Autodesk Inventor part; units mm, degrees
(part 4 of 4)
  arc A540 (15.9898, 14.9832) -> (15.5153, 14.8775) centre (17.401, 7.5282) ccw projected
  arc A541 (15.5153, 14.8775) -> (15.1369, 14.7679) centre (17.1075, 8.6707) ccw projected
  arc A542 (15.1369, 14.7679) -> (14.8419, 14.6628) centre (16.7577, 9.7513) ccw projected
  arc A543 (14.8419, 14.6628) -> (14.619, 14.9696) centre (-0.9435, 3.4284) ccw projected
  arc A544 (14.619, 14.9696) -> (14.8101, 15.2177) centre (10.5399, 18.3094) ccw projected
  arc A545 (14.8101, 15.2177) -> (15.0312, 15.5438) centre (9.6202, 18.976) ccw projected
  arc A546 (15.0312, 15.5438) -> (15.2784, 15.9624) centre (8.6244, 19.6082) ccw projected
  arc A547 (15.2784, 15.9624) -> (15.0311, 16.2761) centre (-0.9435, 3.4284) ccw projected
  arc A548 (15.0311, 16.2761) -> (14.5663, 16.1335) centre (17.0228, 8.9549) ccw projected
  arc A549 (14.5663, 16.1335) -> (14.1976, 15.9946) centre (16.6405, 10.0708) ccw projected
  arc A550 (14.1976, 15.9946) -> (13.9118, 15.8667) centre (16.2071, 11.1207) ccw projected
  arc A551 (13.9118, 15.8667) -> (13.6655, 16.1551) centre (-0.9435, 3.4284) ccw projected
  arc A552 (13.6655, 16.1551) -> (13.8365, 16.4174) centre (9.3369, 19.1645) ccw projected
  arc A553 (13.8365, 16.4174) -> (14.0314, 16.7598) centre (8.3678, 19.7569) ccw projected
  arc A554 (14.0314, 16.7598) -> (14.2449, 17.1965) centre (7.3254, 20.309) ccw projected
  arc A555 (14.2449, 17.1965) -> (13.9738, 17.4899) centre (-0.9435, 3.4284) ccw projected
  arc A556 (13.9738, 17.4899) -> (13.5217, 17.3113) centre (16.5338, 10.3475) ccw projected
  arc A557 (13.5217, 17.3113) -> (13.165, 17.1438) centre (16.0652, 11.43) ccw projected
  arc A558 (13.165, 17.1438) -> (12.8901, 16.9939) centre (15.5507, 12.4426) ccw projected
  arc A559 (12.8901, 16.9939) -> (12.6219, 17.2621) centre (-0.9435, 3.4284) ccw projected
  arc A560 (12.6219, 17.2621) -> (12.7719, 17.537) centre (8.0706, 19.9226) ccw projected
  arc A561 (12.7719, 17.537) -> (12.9393, 17.8936) centre (7.058, 20.4371) ccw projected
  arc A562 (12.9393, 17.8936) -> (13.1179, 18.3458) centre (5.9755, 20.9058) ccw projected
  arc A563 (13.1179, 18.3458) -> (12.8246, 18.6169) centre (-0.9435, 3.4284) ccw projected
  arc A564 (12.8246, 18.6169) -> (12.3878, 18.4034) centre (15.9371, 11.6974) ccw projected
  arc A565 (12.3878, 18.4034) -> (12.0454, 18.2085) centre (15.3849, 12.7398) ccw projected
  arc A566 (12.0454, 18.2085) -> (11.7831, 18.0374) centre (14.7926, 13.7089) ccw projected
  arc A567 (11.7831, 18.0374) -> (11.4947, 18.2837) centre (-0.9435, 3.4284) ccw projected
  arc A568 (11.4947, 18.2837) -> (11.6226, 18.5696) centre (6.7487, 20.579) ccw projected
  arc A569 (11.6226, 18.5696) -> (11.7616, 18.9383) centre (5.6989, 21.0125) ccw projected
  arc A570 (11.7616, 18.9383) -> (11.9041, 19.403) centre (4.5829, 21.3947) ccw projected
  arc A571 (11.9041, 19.403) -> (11.5904, 19.6503) centre (-0.9435, 3.4284) ccw projected
  arc A572 (11.5904, 19.6503) -> (11.1718, 19.4032) centre (15.2362, 12.9963) ccw projected
  arc A573 (11.1718, 19.4032) -> (10.8458, 19.182) centre (14.604, 13.9922) ccw projected
  arc A574 (10.8458, 19.182) -> (10.5977, 18.9909) centre (13.9375, 14.9118) ccw projected
  arc A575 (10.5977, 18.9909) -> (10.2909, 19.2138) centre (-0.9435, 3.4284) ccw projected
  arc A576 (10.2909, 19.2138) -> (10.3959, 19.5089) centre (5.3794, 21.1297) ccw projected
  arc A577 (10.3959, 19.5089) -> (10.5055, 19.8873) centre (4.2988, 21.4794) ccw projected
  arc A578 (10.5055, 19.8873) -> (10.6112, 20.3618) centre (3.1562, 21.773) ccw projected
  arc A579 (10.6112, 20.3618) -> (10.279, 20.5837) centre (-0.9435, 3.4284) ccw projected
  arc A580 (10.279, 20.5837) -> (9.8811, 20.3045) centre (14.4357, 14.2363) ccw projected
  arc A581 (9.8811, 20.3045) -> (9.5734, 20.0585) centre (13.7273, 15.1795) ccw projected
  arc A582 (9.5734, 20.0585) -> (9.3411, 19.8485) centre (12.9906, 16.044) ccw projected
  arc A583 (9.3411, 19.8485) -> (9.0177, 20.0466) centre (-0.9435, 3.4284) ccw projected
  arc A584 (9.0177, 20.0466) -> (9.0993, 20.349) centre (3.971, 21.5712) ccw projected
  arc A585 (9.0993, 20.349) -> (9.1789, 20.7348) centre (2.8663, 21.8351) ccw projected
  arc A586 (9.1789, 20.7348) -> (9.247, 21.2162) centre (1.7043, 22.0381) ccw projected
  arc A587 (9.247, 21.2162) -> (8.8985, 21.4113) centre (-0.9435, 3.4284) ccw projected
  arc A588 (8.8985, 21.4113) -> (8.5237, 21.1018) centre (13.5403, 15.4096) ccw projected
  arc A589 (8.5237, 21.1018) -> (8.2362, 20.8323) centre (12.7601, 16.2943) ccw projected
  arc A590 (8.2362, 20.8323) -> (8.0211, 20.6048) centre (11.9579, 17.0984) ccw projected
  arc A591 (8.0211, 20.6048) -> (7.6832, 20.7769) centre (-0.9435, 3.4284) ccw projected
  arc A592 (7.6832, 20.7769) -> (7.7408, 21.0848) centre (2.5324, 21.9009) ccw projected
  arc A593 (7.7408, 21.0848) -> (7.7898, 21.4757) centre (1.4104, 22.0773) ccw projected
  arc A594 (7.7898, 21.4757) -> (7.82, 21.9609) centre (0.2361, 22.1885) ccw projected
  arc A595 (7.82, 21.9609) -> (7.4572, 22.1281) centre (-0.9435, 3.4284) ccw projected
  arc A596 (7.4572, 22.1281) -> (7.1078, 21.7901) centre (12.5556, 16.5091) ccw projected
  arc A597 (7.1078, 21.7901) -> (6.8424, 21.4989) centre (11.7084, 17.3298) ccw projected
  arc A598 (6.8424, 21.4989) -> (6.6458, 21.2552) centre (10.8456, 18.0685) ccw projected
  arc A599 (6.6458, 21.2552) -> (6.2954, 21.4003) centre (-0.9435, 3.4284) ccw projected
  arc A600 (6.2954, 21.4003) -> (6.3287, 21.7117) centre (1.0724, 22.1166) ccw projected
  arc A601 (6.3287, 21.7117) -> (6.3469, 22.1053) centre (-0.06, 22.2045) ccw projected
  arc A602 (6.3469, 22.1053) -> (6.3389, 22.5913) centre (-1.2395, 22.2232) ccw projected
  arc A603 (6.3389, 22.5913) -> (5.9641, 22.7296) centre (-0.9435, 3.4284) ccw projected
  arc A604 (5.9641, 22.7296) -> (5.6424, 22.3652) centre (11.4877, 17.5279) ccw projected
  arc A605 (5.6424, 22.3652) -> (5.4006, 22.0541) centre (10.5787, 18.2796) ccw projected
  arc A606 (5.4006, 22.0541) -> (5.2237, 21.7957) centre (9.6606, 18.9483) ccw projected
  arc A607 (5.2237, 21.7957) -> (4.863, 21.9129) centre (-0.9435, 3.4284) ccw projected
  arc A608 (4.863, 21.9129) -> (4.8718, 22.2259) centre (-0.4001, 22.2172) ccw projected
  arc A609 (4.8718, 22.2259) -> (4.8591, 22.6197) centre (-1.5359, 22.2159) ccw projected
  arc A610 (4.8591, 22.6197) -> (4.813, 23.1036) centre (-2.7132, 22.142) ccw projected
  arc A611 (4.813, 23.1036) -> (4.4285, 23.212) centre (-0.9435, 3.4284) ccw projected
  arc A612 (4.4285, 23.212) -> (4.1363, 22.8235) centre (10.3432, 18.4597) ccw projected
  arc A613 (4.1363, 22.8235) -> (3.9197, 22.4944) centre (9.378, 19.1379) ccw projected
  arc A614 (3.9197, 22.4944) -> (3.7636, 22.2229) centre (8.4102, 19.7324) ccw projected
  arc A615 (3.7636, 22.2229) -> (3.3949, 22.3115) centre (-0.9435, 3.4284) ccw projected
  arc A616 (3.3949, 22.3115) -> (3.3791, 22.6242) centre (-1.8759, 22.2019) ccw projected
  arc A617 (3.3791, 22.6242) -> (3.3355, 23.0158) centre (-3.0081, 22.1115) ccw projected
  arc A618 (3.3355, 23.0158) -> (3.2515, 23.4946) centre (-4.176, 21.9455) ccw projected
  arc A619 (3.2515, 23.4946) -> (2.8597, 23.5725) centre (-0.9435, 3.4284) ccw projected
  arc A620 (2.8597, 23.5725) -> (2.5989, 23.1623) centre (9.129, 19.299) ccw projected
  arc A621 (2.5989, 23.1623) -> (2.4088, 22.8172) centre (8.1136, 19.8993) ccw projected
  arc A622 (2.4088, 22.8172) -> (2.2745, 22.5343) centre (7.1022, 20.4161) ccw projected
  arc A623 (2.2745, 22.5343) -> (1.9, 22.5936) centre (-0.9435, 3.4284) ccw projected
  arc A624 (1.9, 22.5936) -> (1.8597, 22.9042) centre (-3.346, 22.0709) ccw projected
  arc A625 (1.8597, 22.9042) -> (1.7855, 23.2911) centre (-4.4676, 21.8919) ccw projected
  arc A626 (1.7855, 23.2911) -> (1.6642, 23.7619) centre (-5.6188, 21.6348) ccw projected
  arc A627 (1.6642, 23.7619) -> (1.2675, 23.8088) centre (-0.9435, 3.4284) ccw projected
  arc A628 (1.2675, 23.8088) -> (1.0397, 23.3794) centre (7.8528, 20.0403) ccw projected
  arc A629 (1.0397, 23.3794) -> (0.8773, 23.0205) centre (6.7934, 20.5591) ccw projected
  arc A630 (0.8773, 23.0205) -> (0.7656, 22.7279) centre (5.7445, 20.995) ccw projected
  arc A631 (0.7656, 22.7279) -> (0.3875, 22.7577) centre (-0.9435, 3.4284) ccw projected
  arc A632 (0.3875, 22.7577) -> (0.323, 23.0641) centre (-4.8013, 21.8249) ccw projected
  arc A633 (0.323, 23.0641) -> (0.2187, 23.444) centre (-5.9054, 21.5585) ccw projected
  arc A634 (0.2187, 23.444) -> (0.0608, 23.9038) centre (-7.0329, 21.2118) ccw projected
  arc A635 (0.0608, 23.9038) -> (-0.3383, 23.9195) centre (-0.9435, 3.4284) ccw projected
  arc A636 (-0.3383, 23.9195) -> (-0.5317, 23.4735) centre (6.5223, 20.6793) ccw projected
  arc A637 (-0.5317, 23.4735) -> (-0.6655, 23.1029) centre (5.4255, 21.1133) ccw projected
  arc A638 (-0.6655, 23.1029) -> (-0.7539, 22.8025) centre (4.3457, 21.4655) ccw projected
  arc A639 (-0.7539, 22.8025) -> (-1.1332, 22.8025) centre (-0.9435, 3.4284) ccw projected
  circle A640 centre (-0.9435, 3.4284) radius 18.25
  point P0 (0, 0)
  dimension "d5" = 36.5
  constraints: 1 centre point, 1 coincident
  measures "d5" diameter of A640
extrude "押し出し3" cut sketch "スケッチ3" against normal blind 0.75 contours A640
sketch "スケッチ4" plane through (0.9435, 3.4284, 0.75) normal (0, 0, -1) x (-1, 0, 0)
  circle A0 centre (0, 0) radius 2
  circle A1 centre (0, 0) radius 10.75
  arc A2 (0.7009, 4.7673) -> (0.6658, 4.6511) centre (1.2537, 4.5366) ccw
  arc A3 (0.9055, 5.1323) -> (0.7009, 4.7673) centre (2.2508, 4.1383) ccw
  arc A4 (1.5725, 5.7903) -> (0.9055, 5.1323) centre (3.314, 3.3579) ccw
  arc A5 (-2.2351, 4.2688) -> (-2.1952, 4.1541) centre (-1.6522, 4.4071) ccw
  arc A6 (-2.2841, 4.6844) -> (-2.2351, 4.2688) centre (-0.6115, 4.671) ccw
  arc A7 (-2.1312, 5.6087) -> (-2.2841, 4.6844) centre (0.7074, 4.6645) ccw
  arc A8 (-4.3174, 2.1398) -> (-4.2177, 2.0704) centre (-3.9271, 2.5942) ccw
  arc A9 (-4.6013, 2.4472) -> (-4.3174, 2.1398) centre (-3.2402, 3.4195) ccw
  arc A10 (-5.0209, 3.2848) -> (-4.6013, 2.4472) centre (-2.1695, 4.1895) ccw
  arc A11 (-4.7506, -0.8065) -> (-4.6291, -0.8041) centre (-4.7019, -0.2095) ccw
  arc A12 (-5.1609, -0.7247) -> (-4.7506, -0.8065) centre (-4.6313, 0.8619) ccw
  arc A13 (-5.9928, -0.2937) -> (-5.1609, -0.7247) centre (-4.2177, 2.1142) ccw
  arc A14 (-3.3692, -3.4448) -> (-3.2724, -3.3715) centre (-3.6808, -2.9332) ccw
  arc A15 (-3.7493, -3.6198) -> (-3.3692, -3.4448) centre (-4.2534, -2.025) ccw
  arc A16 (-4.6756, -3.7601) -> (-3.7493, -3.6198) centre (-4.6548, -0.7687) ccw
  arc A17 (-0.7009, -4.7673) -> (-0.6658, -4.6511) centre (-1.2537, -4.5366) ccw
  arc A18 (-0.9055, -5.1323) -> (-0.7009, -4.7673) centre (-2.2508, -4.1383) ccw
  arc A19 (-1.5725, -5.7903) -> (-0.9055, -5.1323) centre (-3.314, -3.3579) ccw
  arc A20 (2.2351, -4.2688) -> (2.1952, -4.1541) centre (1.6522, -4.4071) ccw
  arc A21 (2.2841, -4.6791) -> (2.2351, -4.2688) centre (0.6115, -4.671) ccw
  arc A22 (2.1312, -5.6087) -> (2.2841, -4.6791) centre (-0.7074, -4.6645) ccw
  arc A23 (4.3174, -2.1398) -> (4.2177, -2.0704) centre (3.9271, -2.5942) ccw
  arc A24 (4.6013, -2.4472) -> (4.3174, -2.1398) centre (3.2402, -3.4195) ccw
  arc A25 (5.0209, -3.2848) -> (4.6013, -2.4472) centre (2.1695, -4.1895) ccw
  arc A26 (4.7506, 0.8065) -> (4.6291, 0.8041) centre (4.7019, 0.2095) ccw
  arc A27 (5.1609, 0.7247) -> (4.7506, 0.8065) centre (4.6313, -0.8619) ccw
  arc A28 (5.9928, 0.2937) -> (5.1609, 0.7247) centre (4.2177, -2.1142) ccw
  arc A29 (3.3692, 3.4448) -> (3.2724, 3.3715) centre (3.6808, 2.9332) ccw
  arc A30 (3.7493, 3.6198) -> (3.3692, 3.4448) centre (4.2534, 2.025) ccw
  arc A31 (4.6756, 3.7601) -> (3.7493, 3.6198) centre (4.6548, 0.7687) ccw
  arc A32 (-0.6658, 4.6511) -> (-0.7009, 4.7673) centre (-1.2537, 4.5366) ccw
  arc A33 (-0.7009, 4.7673) -> (-0.9055, 5.1323) centre (-2.2508, 4.1383) ccw
  arc A34 (-0.9055, 5.1323) -> (-1.5725, 5.7903) centre (-3.314, 3.3579) ccw
  arc A35 (-3.2724, 3.3715) -> (-3.3692, 3.4448) centre (-3.6808, 2.9332) ccw
  arc A36 (-3.3692, 3.4448) -> (-3.7493, 3.6198) centre (-4.2534, 2.025) ccw
  arc A37 (-3.7493, 3.6198) -> (-4.6756, 3.7601) centre (-4.6548, 0.7687) ccw
  arc A38 (-4.6291, 0.8041) -> (-4.7506, 0.8065) centre (-4.7019, 0.2095) ccw
  arc A39 (-4.7506, 0.8065) -> (-5.1609, 0.7247) centre (-4.6313, -0.8619) ccw
  arc A40 (-5.1609, 0.7247) -> (-5.9928, 0.2937) centre (-4.2177, -2.1142) ccw
  arc A41 (-4.2177, -2.0704) -> (-4.3174, -2.1398) centre (-3.9271, -2.5942) ccw
  arc A42 (-4.3174, -2.1398) -> (-4.6013, -2.4472) centre (-3.2402, -3.4195) ccw
  arc A43 (-4.6013, -2.4472) -> (-5.0209, -3.2848) centre (-2.1695, -4.1895) ccw
  arc A44 (-2.1952, -4.1541) -> (-2.2351, -4.2688) centre (-1.6522, -4.4071) ccw
  arc A45 (-2.2351, -4.2688) -> (-2.2841, -4.6844) centre (-0.6115, -4.671) ccw
  arc A46 (-2.2841, -4.6844) -> (-2.1312, -5.6087) centre (0.7074, -4.6645) ccw
  arc A47 (0.6658, -4.6511) -> (0.7009, -4.7673) centre (1.2537, -4.5366) ccw
  arc A48 (0.7009, -4.7673) -> (0.9024, -5.128) centre (2.2508, -4.1383) ccw
  arc A49 (0.9024, -5.128) -> (1.5725, -5.7903) centre (3.314, -3.3579) ccw
  arc A50 (3.2724, -3.3715) -> (3.3692, -3.4448) centre (3.6808, -2.9332) ccw
  arc A51 (3.3692, -3.4448) -> (3.7493, -3.6198) centre (4.2534, -2.025) ccw
  arc A52 (3.7493, -3.6198) -> (4.6756, -3.7601) centre (4.6548, -0.7687) ccw
  arc A53 (4.6291, -0.8041) -> (4.7506, -0.8065) centre (4.7019, -0.2095) ccw
  arc A54 (4.7506, -0.8065) -> (5.1609, -0.7247) centre (4.6313, 0.8619) ccw
  arc A55 (5.1609, -0.7247) -> (5.9928, -0.2937) centre (4.2177, 2.1142) ccw
  arc A56 (4.2177, 2.0704) -> (4.3174, 2.1398) centre (3.9271, 2.5942) ccw
  arc A57 (4.3174, 2.1398) -> (4.6013, 2.4472) centre (3.2402, 3.4195) ccw
  arc A58 (4.6013, 2.4472) -> (5.0209, 3.2848) centre (2.1695, 4.1895) ccw
  arc A59 (2.1952, 4.1541) -> (2.2351, 4.2688) centre (1.6522, 4.4071) ccw
  arc A60 (2.2351, 4.2688) -> (2.2841, 4.6844) centre (0.6115, 4.671) ccw
  arc A61 (2.2841, 4.6844) -> (2.1312, 5.6087) centre (-0.7074, 4.6645) ccw
  arc A62 (0.5314, 3.7122) -> (-0.5314, 3.7122) centre (0, 0) ccw
  arc A63 (-1.7521, 3.3155) -> (-2.6118, 2.6909) centre (0, 0) ccw
  arc A64 (-3.3663, 1.6525) -> (-3.6947, 0.6418) centre (0, 0) ccw
  arc A65 (-3.6947, -0.6418) -> (-3.3663, -1.6525) centre (0, 0) ccw
  arc A66 (-2.6118, -2.6909) -> (-1.7521, -3.3155) centre (0, 0) ccw
  arc A67 (-0.5314, -3.7122) -> (0.5314, -3.7122) centre (0, 0) ccw
  arc A68 (1.7521, -3.3155) -> (2.6118, -2.6909) centre (0, 0) ccw
  arc A69 (3.3663, -1.6525) -> (3.6947, -0.6418) centre (0, 0) ccw
  arc A70 (3.6947, 0.6418) -> (3.3663, 1.6525) centre (0, 0) ccw
  arc A71 (2.6118, 2.6909) -> (1.7521, 3.3155) centre (0, 0) ccw
  arc A72 (-1.5725, 5.7903) -> (-2.1312, 5.6087) centre (0, 0) ccw
  arc A73 (-4.6756, 3.7601) -> (-5.0209, 3.2848) centre (0, 0) ccw
  arc A74 (-5.9928, 0.2937) -> (-5.9928, -0.2937) centre (0, 0) ccw
  arc A75 (-5.0209, -3.2848) -> (-4.6756, -3.7601) centre (0, 0) ccw
  arc A76 (-2.1312, -5.6087) -> (-1.5725, -5.7903) centre (0, 0) ccw
  arc A77 (1.5725, -5.7903) -> (2.1312, -5.6087) centre (0, 0) ccw
  arc A78 (4.6756, -3.7601) -> (5.0209, -3.2848) centre (0, 0) ccw
  arc A79 (5.9928, -0.2937) -> (5.9928, 0.2937) centre (0, 0) ccw
  arc A80 (5.0209, 3.2848) -> (4.6756, 3.7601) centre (0, 0) ccw
  arc A81 (2.1312, 5.6087) -> (1.5725, 5.7903) centre (0, 0) ccw
  line L0 (0.5314, 3.7122) -> (0.6658, 4.6511)
  line L1 (-1.7521, 3.3155) -> (-2.1952, 4.1541)
  line L2 (-3.3663, 1.6525) -> (-4.2177, 2.0704)
  line L3 (-3.6947, -0.6418) -> (-4.6291, -0.8041)
  line L4 (-2.6118, -2.6909) -> (-3.2724, -3.3715)
  line L5 (-0.5314, -3.7122) -> (-0.6658, -4.6511)
  line L6 (1.7521, -3.3155) -> (2.1952, -4.1541)
  line L7 (3.3663, -1.6525) -> (4.2177, -2.0704)
  line L8 (3.6947, 0.6418) -> (4.6291, 0.8041)
  line L9 (2.6118, 2.6909) -> (3.2724, 3.3715)
  line L10 (-0.5314, 3.7122) -> (-0.6658, 4.6511)
  line L11 (-2.6118, 2.6909) -> (-3.2724, 3.3715)
  line L12 (-3.6947, 0.6418) -> (-4.6291, 0.8041)
  line L13 (-3.3663, -1.6525) -> (-4.2177, -2.0704)
  line L14 (-1.7521, -3.3155) -> (-2.1952, -4.1541)
  line L15 (0.5314, -3.7122) -> (0.6658, -4.6511)
  line L16 (2.6118, -2.6909) -> (3.2724, -3.3715)
  line L17 (3.6947, -0.6418) -> (4.6291, -0.8041)
  line L18 (3.3663, 1.6525) -> (4.2177, 2.0704)
  line L19 (1.7521, 3.3155) -> (2.1952, 4.1541)
  line L20 (-8, 0) -> (8, 0)
  line L21 (0, -8) -> (0, 8)
  line L22 (19.1279, 81.4836) -> (89.1279, 81.4836)
  line L23 (19.1279, 73.4836) -> (89.1279, 73.4836)
  line L24 (19.1279, 65.4836) -> (89.1279, 65.4836)
  line L25 (19.1279, 57.4836) -> (89.1279, 57.4836)
  line L26 (19.1279, 49.4836) -> (89.1279, 49.4836)
  line L27 (19.1279, 41.4836) -> (89.1279, 41.4836)
  line L28 (19.1279, 33.4836) -> (89.1279, 33.4836)
  line L29 (19.1279, 25.4836) -> (89.1279, 25.4836)
  line L30 (19.1279, 17.4836) -> (89.1279, 17.4836)
  line L31 (19.1279, 9.4836) -> (89.1279, 9.4836)
  line L32 (19.1279, 1.4836) -> (89.1279, 1.4836)
  line L33 (19.1279, -6.5164) -> (89.1279, -6.5164)
  line L34 (19.1279, -14.5164) -> (89.1279, -14.5164)
  line L35 (19.1279, 81.4836) -> (19.1279, -14.5164)
  line L36 (89.1279, 81.4836) -> (89.1279, -14.5164)
  line L37 (54.1279, 73.4836) -> (54.1279, -14.5164)
  point P0 (0.9435, -3.4284)
  point P1 (7.5077, -72.712)
  point P2 (25.1279, 75.4836)
  point P3 (27.6279, 67.4836)
  point P4 (27.6279, 59.4836)
  point P5 (25.1279, 51.4836)
  point P6 (27.6279, 43.4836)
  point P7 (22.6279, 35.4836)
  point P8 (25.1279, 27.4836)
  point P9 (25.1279, 19.4836)
  point P10 (25.1279, 11.4836)
  point P11 (27.6279, 3.4836)
  point P12 (27.6279, -4.5164)
  point P13 (25.1279, -12.5164)
  point P14 (55.1279, 67.4836)
  point P15 (70.1279, 59.4836)
  point P16 (71.3779, 51.4836)
  point P17 (67.6279, 43.4836)
  point P18 (70.1279, 35.4836)
  point P19 (65.1279, 27.4836)
  point P20 (70.1279, 19.4836)
  point P21 (68.8779, 11.4836)
  point P22 (65.1279, 3.4836)
  point P23 (-5.8721, 96.9836)
  point P24 (-5.8721, 90.9836)
  point P25 (12.4404, 96.9836)
  point P26 (13.5029, 90.9836)
  constraints: 160 point on circle, 82 centre point, 72 end point, 2 midpoint, 53 other
extrude "押し出し4" add sketch "スケッチ4" along normal blind 5.75 contours L20 A79 A55 A54 A53 L17 A69 L7 A23 A24 A25 A78 A52 A51 A50 L16 A68 L6 A20 A21 A22 A77 A49 A48 A47 L15 A67 L21 A0 | A0 L21 A62 L0 A2 A3 A4 A81 A61 A60 A59 L19 A71 L9 A29 A30 A31 A80 A58 A57 A56 L18 A70 L8 A26 A27 A28 A79 L20 | A0 L20 A74 A40 A39 A38 L12 A64 L2 A8 A9 A10 A73 A37 A36 A35 L11 A63 L1 A5 A6 A7 A72 A34 A33 A32 L10 A62 L21 | L21 A67 L5 A17 A18 A19 A76 A46 A45 A44 L14 A66 L4 A14 A15 A16 A75 A43 A42 A41 L13 A65 L3 A11 A12 A13 A74 L20 A0
sketch "スケッチ5" plane through (0.9435, 3.4284, 0.75) normal (0, 0, -1) x (-1, 0, 0)
  circle A0 centre (0, 0) radius 2 projected
  point P0 (0.9435, -3.4284)
extrude "押し出し5" cut sketch "スケッチ5" against normal blind 10
sketch "スケッチ6" plane through (0.9435, 3.4284, 2.25) normal (0, 0, 1) x (1, 0, 0)
  circle A0 centre (0, 0) radius 2 projected
  circle A1 centre (0, 0) radius 6
  point P0 (-0.9435, -3.4284)
  dimension "d12" = 12
  constraints: 1 centre point, 1 coincident
  measures "d12" diameter of A1
extrude "押し出し6" add sketch "スケッチ6" along normal blind 0.75
chamfer "面取り1" distance 0.25 angle 45 1 edges at (-5.0565, 3.4284, 3)
sketch "スケッチ11" plane through (0.9435, 3.4284, 2.25) normal (0, 0, 1) x (1, 0, 0)
  circle A0 centre (0, 0) radius 18.25 projected
  circle A1 centre (0, 0) radius 6 projected
  circle A2 centre (0, 0) radius 14.25
  circle A3 centre (0, 0) radius 9
  line L0 (-18.25, 0) -> (18.25, 0)
  line L1 (0, -18.25) -> (0, 18.25)
  line L2 (-1.5, 14.1708) -> (-2, 8.775)
  line L3 (1.5, 14.1708) -> (2, 8.775)
  line L4 (8.775, 2) -> (14.1708, 1.5)
  line L5 (8.775, -2) -> (14.1708, -1.5)
  line L6 (2, -8.775) -> (1.5, -14.1708)
  line L7 (-1.5, -14.1708) -> (-2, -8.775)
  line L8 (-14.1708, -1.5) -> (-8.775, -2)
  line L9 (-14.1708, 1.5) -> (-8.775, 2)
  point P0 (-0.9435, -3.4284)
  dimension "d46" = 4
  dimension "d47" = 3
  dimension "d48" = 1.5
  dimension "d49" = 1.5
  dimension "d50" = 1.5
  dimension "d51" = 1.5
  dimension "d52" = 1.5
  dimension "d53" = 1.5
  dimension "d54" = 1.5
  dimension "d55" = 1.5
  dimension "d56" = 2
  dimension "d57" = 2
  dimension "d58" = 2
  dimension "d59" = 2
  dimension "d60" = 2
  dimension "d61" = 2
  dimension "d62" = 2
  dimension "d63" = 2
  constraints: 20 end point, 4 point on circle, 2 midpoint, 1 coincident, 1 horizontal, 1 vertical, 20 other
  measures "d48" distance from line of L1 L2.start
  measures "d49" distance from line of L3.start L1
  measures "d50" distance from line of L0 L4.end
  measures "d51" distance from line of L0 L5.end
  measures "d52" distance from line of L1 L6.end
  measures "d53" distance from line of L1 L7.start
  measures "d54" distance from line of L0 L9.start
  measures "d55" distance from line of L8.start L0
  measures "d56" distance from line of L1 L2.end
  measures "d57" distance from line of L1 L3.end
  measures "d58" distance from line of L0 L4.start
  measures "d59" distance from line of L0 L5.start
  measures "d60" distance from line of L1 L6.start
  measures "d61" distance from line of L1 L7.end
  measures "d62" distance from line of L0 L8.end
  measures "d63" distance from line of L0 L9.end
extrude "押し出し10" cut sketch "スケッチ11" against normal through all contours L4 A3 L3 A2 | A2 L6 A3 L5 | L2 A3 L9 A2 | A2 L8 A3 L7
fillet "フィレット2" radius 2 16 edges at (9.7185, 5.4284, 1.5) (9.7185, 1.4284, 1.5) (15.1144, 1.9284, 1.5) (15.1144, 4.9284, 1.5) (-0.5565, 17.5993, 1.5) (-1.0565, 12.2034, 1.5) (2.9435, 12.2034, 1.5) (2.4435, 17.5993, 1.5) (-7.8314, 5.4284, 1.5) (-7.8314, 1.4284, 1.5) (-13.2273, 4.9284, 1.5) (-13.2273, 1.9284, 1.5) (-1.0565, -5.3465, 1.5) (2.9435, -5.3465, 1.5) (2.4435, -10.7424, 1.5) (-0.5565, -10.7424, 1.5)
equation "\"d49\" = d48"
equation "\"d50\" = d49"
equation "\"d51\" = d50"
equation "\"d52\" = d51"
equation "\"d53\" = d52"
equation "\"d54\" = d48"
